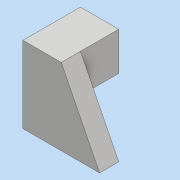
# Autodesk Inventor part: 3
Saved by Autodesk Inventor 2017 (Build 210142000, 142)
## iProperties
Part Number: 3
Material: 一般
Document SubType Name: Modeling
Designer: d8910
Density: 1 g/cm^3
Appearance: 預設
Author: d8910
Autodesk Inventor part; units mm, degrees
ref_plane "YZ Plane" through (0, 0, 0) normal (1, 0, 0) x (0, 1, 0)
ref_plane "XZ Plane" through (0, 0, 0) normal (0, 1, 0) x (-1, 0, 0)
ref_plane "XY Plane" through (0, 0, 0) normal (0, 0, 1) x (1, 0, 0)
sketch "草圖1" plane through (0, 0, 0) normal (0, 1, 0) x (-1, 0, 0)
  line L0 (10, 10) -> (0, 10)
  line L1 (-10, 10) -> (-10, -10) construction
  line L2 (-10, -10) -> (10, -10)
  line L3 (10, -10) -> (10, 10)
  line L4 (10, 10) -> (0, 10)
  line L5 (0, 10) -> (0, 0)
  line L6 (0, 0) -> (10, 0)
  line L7 (10, 0) -> (10, 10)
  line L8 (0, 10) -> (-10, -10)
  line L9 (0, 10) -> (-10, 10) construction
  point P0 (0, -10)
  point P1 (10, 0)
  dimension "d0" = 20
  constraints: 20 end point, 5 parallel, 4 perpendicular, 3 horizontal, 2 midpoint, 1 horizontal alignment, 1 vertical alignment
  measures "d0" distance of L2.end L0.start
extrude "擠出1" add sketch "草圖1" along normal blind 5 contours L5 L6 L3 L2 L8
extrude "擠出2" add sketch "草圖1" along normal blind 15 contours L3 L6 L5 L0
